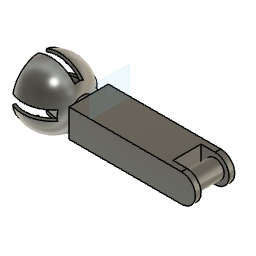
first_joint_bs v7 (Autodesk Fusion 360 design; units mm, degrees)
Autodesk Fusion 360 part; units mm, degrees
note: some values were not read from the file. Chosen so that the rebuilt part matches the saved one: which bodies a step acts on. Set by a fixed rule: which sketch regions a step uses.
sketch "Sketch1" plane through (0, 0, 0) normal (0, 1, 0) x (1, 0, 0)
  circle A0 centre (0, 0) radius 5
  line L0 (0, -5) -> (40, -5)
  line L1 (40, -5) -> (40, 5)
  line L2 (40, 5) -> (0, 5)
  line L3 (0, 5) -> (0, -5)
  line L4 (20, -5) -> (22.5, -5)
  line L5 (22.5, -5) -> (22.5, -15)
  line L6 (22.5, -15) -> (20, -15)
  line L7 (20, -15) -> (20, -5)
  dimension "d1" = 10
  dimension "d2" = 40
  dimension "d3" = 2.5
  dimension "d4" = 10
  dimension "d5" = 20
  constraint coincident A0.centre origin
  constraint horizontal L0
  constraint vertical L1
  constraint horizontal L2
  constraint vertical L3
  constraint coincident A0 L0.start
  constraint horizontal L4
  constraint vertical L5
  constraint horizontal L6
  constraint vertical L7
  constraint coincident L0 L4.start
  measures "d1" diameter of A0
  measures "d2" distance of L0.start L0.end
  measures "d3" distance of L4.start L4.end
  measures "d4" distance of L4.start L6.end
  measures "d5" distance of A0.centre L7
extrude "Extrude1" add sketch "Sketch1" along normal blind 14 makes body 1
sketch "Sketch2" plane through (0, 0, 5) normal (0, 0, 1) x (-1, 0, 0)
  line L0 (0, 0) -> (-20, 0)
  line L1 (-20, 0) -> (-20, -14)
  line L2 (-20, -14) -> (0, -14)
  line L3 (0, -14) -> (0, 0)
  line L4 (-5, -12) -> (5, -12)
  line L5 (5, -12) -> (5, -2)
  line L6 (5, -2) -> (-5, -2)
  line L7 (-5, -2) -> (-5, -12)
  dimension "d8" = 10
  dimension "d9" = 10
  dimension "d10" = 25
  constraint horizontal L4
  constraint vertical L5
  constraint horizontal L6
  constraint vertical L7
  measures "d8" distance of L4.start L4.end
  measures "d9" distance of L4.start L6.end
  measures "d10" distance of L1 L5
extrude "Extrude2" cut sketch "Sketch2" against normal blind 50 contours L3 L4 L5 L6 | L3 L4 L6 L7 bodies 1
sketch "Sketch3" plane through (0, 0, 0) normal (0, -1, 0) x (1, 0, 0)
  line L0 (40, 5) -> (22.5, 5)
  line L1 (22.5, 5) -> (22.5, 15)
  line L2 (22.5, 15) -> (20, 15)
  line L3 (20, 15) -> (20, 5)
  line L4 (20, 5) -> (0, 5)
  arc A0 (0, 5) -> (0, -5) centre (0, 0) ccw
  line L5 (0, -5) -> (40, -5)
  line L6 (40, -5) -> (40, 5)
  circle A1 centre (0, 0) radius 1.5
  dimension "d13" = 3
  constraint coincident A0.centre A1.centre
  measures "d13" diameter of A1
extrude "Extrude3" cut sketch "Sketch3" against normal blind 22 contours A1 bodies 1
sketch "Sketch4" plane through (22.5, 0, 0) normal (1, 0, 0) x (0, 1, 0)
  line L0 (0, 15) -> (0, 5)
  line L1 (0, 5) -> (14, 5)
  line L2 (14, 5) -> (14, 15)
  line L3 (14, 15) -> (0, 15)
  circle A0 centre (7, 10) radius 1
  dimension "d16" = 2
  measures "d16" diameter of A0
extrude "Extrude4" cut sketch "Sketch4" against normal blind 46 contours A0 bodies 1
sketch "Sketch5" plane through (40, 0, 0) normal (1, 0, 0) x (0, 1, 0)
  line L0 (0, 5) -> (0, -5)
  line L1 (0, -5) -> (14, -5)
  line L2 (14, -5) -> (14, 5)
  line L3 (14, 5) -> (0, 5)
  line L4 (0, 5) -> (14, 5)
  line L5 (14, 5) -> (14, -5)
  line L6 (14, -5) -> (0, -5)
  line L7 (0, -5) -> (0, 5)
  constraint horizontal L4
  constraint vertical L5
  constraint horizontal L6
  constraint vertical L7
  constraint coincident L1.end L2.start
  constraint coincident L0.start L3.end
extrude "Extrude5" add sketch "Sketch5" along normal blind 20 bodies 1
fillet "Fillet1" radius 5 2 edges at (60, 7, 5) (60, 7, -5) on bodies 1
sketch "Sketch6" plane through (0, 0, 5) normal (0, 0, 1) x (-1, 0, 0)
  line L0 (-55, 0) -> (-55, -14)
  line L1 (-55, -14) -> (-22.5, -14)
  line L2 (-22.5, -14) -> (-22.5, 0)
  line L3 (-22.5, 0) -> (-55, 0)
  line L4 (-60, -12) -> (-50, -12)
  line L5 (-50, -12) -> (-50, -2)
  line L6 (-50, -2) -> (-60, -2)
  line L7 (-60, -2) -> (-60, -12)
  dimension "d23" = 10
  dimension "d24" = 10
  constraint horizontal L4
  constraint vertical L5
  constraint horizontal L6
  constraint vertical L7
  measures "d23" distance of L4.start L4.end
  measures "d24" distance of L4.start L6.end
extrude "Extrude6" cut sketch "Sketch6" against normal blind 40 contours L0 L4 L5 L6 | L0 L4 L6 L7 bodies 1
sketch "Sketch7" plane through (0, 0, 0) normal (0, -1, 0) x (1, 0, 0)
  circle A0 centre (0, 0) radius 1.5
  arc A1 (55, -5) -> (55, 5) centre (55, 0) ccw
  line L0 (55, 5) -> (22.5, 5)
  line L1 (22.5, 5) -> (22.5, 15)
  line L2 (22.5, 15) -> (20, 15)
  line L3 (20, 15) -> (20, 5)
  line L4 (20, 5) -> (0, 5)
  arc A2 (0, 5) -> (0, -5) centre (0, 0) ccw
  line L5 (0, -5) -> (55, -5)
  circle A3 centre (55, 0) radius 1.5
  dimension "d27" = 3
  constraint concentric A1 A3
  measures "d27" diameter of A3
extrude "Extrude7" cut sketch "Sketch7" against normal blind 44 contours A3 bodies 1
sketch "Sketch8" plane through (0, 0, 0) normal (0, 1, 0) x (1, 0, 0)
sketch "Sketch9" plane through (22.5, 0, 0) normal (1, 0, 0) x (0, 1, 0)
  circle A0 centre (7, 10) radius 1
  line L0 (0, 15) -> (0, 5)
  line L1 (0, 5) -> (14, 5)
  line L2 (14, 5) -> (14, 15)
  line L3 (14, 15) -> (0, 15)
ref_plane "WorkPlane1" through (5, 7, 0) normal (-1, 0, 0) x (0, 1, 0)
sketch "Sketch10" plane through (5, 7, 0) normal (-1, 0, 0) x (0, 1, 0)
  line L0 (7, -5) -> (-7, -5)
  line L1 (-7, -5) -> (-7, 5)
  line L2 (-7, 5) -> (7, 5)
  line L3 (7, 5) -> (7, -5)
  constraint horizontal L0
  constraint vertical L1
  constraint horizontal L2
  constraint vertical L3
extrude "Extrude8" cut sketch "Sketch10" along normal blind 10 bodies 1
sketch "Sketch11" plane through (5, 0, 0) normal (-1, 0, 0) x (0, -1, 0)
  line L0 (-14, -5) -> (0, -5)
  line L1 (0, -5) -> (0, 5)
  line L2 (0, 5) -> (-14, 5)
  line L3 (-14, 5) -> (-14, -5)
  line L4 (-14, 5) -> (0, 5)
  line L5 (0, 5) -> (0, -5)
  line L6 (0, -5) -> (-14, -5)
  line L7 (-14, -5) -> (-14, 5)
  constraint horizontal L4
  constraint vertical L5
  constraint horizontal L6
  constraint vertical L7
  constraint coincident L0.end L1.start
  constraint coincident L2.end L3.start
extrude "Extrude9" cut sketch "Sketch11" against normal blind 10 bodies 1
sketch "Sketch12" plane through (15, 0, 0) normal (-1, 0, 0) x (0, -1, 0)
  line L0 (-14, -5) -> (0, -5)
  line L1 (0, -5) -> (0, 5)
  line L2 (0, 5) -> (-14, 5)
  line L3 (-14, 5) -> (-14, -5)
  circle A0 centre (-7, 0) radius 4
  dimension "d35" = 8
  measures "d35" diameter of A0
extrude "Extrude10" add sketch "Sketch12" along normal blind 12.5 contours A0 bodies 1
ref_plane "WorkPlane2" through (2.5, 7, 0) normal (-1, 0, 0) x (0, -1, 0)
sphere "SpherePrimitive1" add diameter 22.23 placed x (0, 1, 0) y (0, 0, -1) z (-1, 0, 0) at (2.5, 7, 0) separate body makes body 2
ref_plane "WorkPlane3" through (-2, 7, 0) normal (-1, 0, 0) x (0, 0, 1)
sketch "Sketch14" plane through (-2, 7, 0) normal (-1, 0, 0) x (0, 1, 0)
  line L0 (16.9158, -10.9335) -> (-15.7784, -10.9335)
  line L1 (-15.7784, -10.9335) -> (-15.7784, 11.053)
  line L2 (-15.7784, 11.053) -> (16.9158, 11.053)
  line L3 (16.9158, 11.053) -> (16.9158, -10.9335)
  constraint horizontal L0
  constraint vertical L1
  constraint horizontal L2
  constraint vertical L3
extrude "Extrude11" cut sketch "Sketch14" along normal blind 10 bodies 2
copy_body "CopyPasteBodies1" bodies 2 makes body 3
move_body "Move1" bodies 3 to x (1, 0, 0) y (0, 1, 0) z (0, 0, 1) at (-24, 0, 0)
scale "Scale1" factor 0.9 about (-26, 7, -10.1633) bodies 3
move_body "Move2" bodies 3 to x (1, 0, 0) y (0, 1, 0) z (0, 0, 1) at (24, 0, 1.0163)
combine "Combine1" operation add target body 2 tool bodies 1
split "Split1" by bodies 3 bodies 2 makes body 4 at (3.1169, 11.5139, 10.1384)
move_body "Move3" bodies 3 to x (1, 0, 0) y (0, 1, 0) z (0, 0, 1) at (-30, 0, 0)
move_body "Move4" bodies 2 to x (1, 0, 0) y (0, 1, 0) z (0, 0, 1) at (0, 30, 0)
sketch "Sketch18" plane through (0, 14, 0) normal (0, 1, 0) x (-1, 0, 0)
  line L0 (-15, -5) -> (-15, 5)
  line L1 (-15, 5) -> (-20, 5)
  line L2 (-20, 5) -> (-20, 15)
  line L3 (-20, 15) -> (-22.5, 15)
  line L4 (-22.5, 15) -> (-22.5, 5)
  line L5 (-22.5, 5) -> (-55, 5)
  arc A0 (-55, 5) -> (-55, -5) centre (-55, 0) ccw
  line L6 (-55, -5) -> (-15, -5)
  circle A1 centre (-55, 0) radius 1.5
  circle A2 centre (-55, 0) radius 3.25
  dimension "d44" = 6.5
  constraint concentric A0 A2
  measures "d44" diameter of A2
extrude "Extrude12" add sketch "Sketch18" against normal blind 14 contours A1 | A2 bodies 4
sketch "Sketch20" plane through (0, 0, 15) normal (0, 0, 1) x (-1, 0, 0)
  line L0 (-20, 0) -> (-22.5, 0)
  line L1 (-22.5, 0) -> (-22.5, -14)
  line L2 (-22.5, -14) -> (-20, -14)
  line L3 (-20, -14) -> (-20, 0)
  line L4 (2, -9) -> (-11, -9)
  line L5 (-11, -9) -> (-11, -6)
  line L6 (-11, -6) -> (2, -6)
  line L7 (2, -6) -> (2, -9)
  constraint horizontal L4
  constraint vertical L5
  constraint horizontal L6
  constraint vertical L7
extrude "Extrude13" cut sketch "Sketch20" against normal blind 27 contours L4 L5 L6 L7 bodies 4
ref_plane "WorkPlane4" through (37.5, -8, 5) normal (0, -1, 0) x (-1, 0, 0)
sketch "Sketch21" plane through (37.5, -8, 5) normal (0, -1, 0) x (1, 0, 0)
  line L0 (-40, -3) -> (-26.5473, -3)
  line L1 (-26.5473, -3) -> (-26.5473, -6.4628)
  line L2 (-26.5473, -6.4628) -> (-40, -6.4628)
  line L3 (-40, -6.4628) -> (-40, -3)
  constraint horizontal L0
  constraint vertical L1
  constraint horizontal L2
  constraint vertical L3
extrude "Extrude14" cut sketch "Sketch21" against normal blind 70 bodies 4
sketch "Sketch22" plane through (22.5, 0, 0) normal (1, 0, 0) x (0, 1, 0)
  line L0 (-1, 15) -> (16, 15)
  line L1 (16, 15) -> (16, 5)
  line L2 (16, 5) -> (-1, 5)
  line L3 (-1, 5) -> (-1, 15)
  constraint horizontal L0
  constraint vertical L1
  constraint horizontal L2
  constraint vertical L3
extrude "Extrude15" cut sketch "Sketch22" against normal blind 5 bodies 4
hidden bodies 2 3
named bodies: "Socket_Joint", "Ball", "Socket_Joint (1)"
